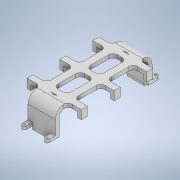
# Autodesk Inventor part: Battery_holder
Saved by Autodesk Inventor 2022 (Build 260153000, 153)
## iProperties
Created: 2023-01-27
Part Number: Battery_holder
Material: Generic
Document SubType Name: Modeling
Designer: Harmonic Ash
Density: 1 g/cm^3
Appearance: Default
Author: Harmonic Ash
Autodesk Inventor part; units mm, degrees
ref_plane "YZ Plane" through (0, 0, 0) normal (1, 0, 0) x (0, 1, 0)
ref_plane "XZ Plane" through (0, 0, 0) normal (0, 1, 0) x (-1, 0, 0)
ref_plane "XY Plane" through (0, 0, 0) normal (0, 0, 1) x (1, 0, 0)
sketch "Sketch1" plane through (0, 0, 0) normal (0, 1, 0) x (-1, 0, 0)
  line L0 (7.7, 0) -> (7.7, 36.5)
  circle A0 centre (7.7, 36.5) radius 0.75
  line L1 (6.2, 30.5) -> (6.2, 36.5)
  circle A1 centre (5.2, 31.5) radius 1
  line L2 (6.2, 30.5) -> (0, 30.5)
  line L3 (0, 30.5) -> (0, 36.5)
  line L4 (0, 36.5) -> (6.2, 36.5)
  line L5 (6.2, 36.5) -> (6.2, 30.5)
  line L6 (7.7, 36.5) -> (0, 36.5)
  line L7 (0, 36.5) -> (0, 0)
  line L8 (0, 0) -> (7.7, 0)
  line L9 (7.7, 0) -> (7.7, 36.5)
  circle A2 centre (7.7, 36.5) radius 1.5
  line L10 (9.2, 36.5) -> (7.7, 36.5)
  line L11 (7.7, 36.5) -> (7.7, 0)
  line L12 (7.7, 0) -> (9.2, 0)
  line L13 (9.2, 0) -> (9.2, 36.5)
  line L14 (6.2, 30.5) -> (0, 30.5)
  line L15 (0, 30.5) -> (0, 33)
  line L16 (0, 33) -> (6.2, 33)
  line L17 (6.2, 33) -> (6.2, 30.5)
  line L18 (9.5, 16) -> (6.5, 16)
  line L19 (6.5, 16) -> (6.5, 0)
  line L20 (6.5, 0) -> (9.5, 0)
  line L21 (9.5, 0) -> (9.5, 16)
  circle A3 centre (8, 16) radius 1.5
  line L22 (0, 0) -> (12.5, 0)
  line L23 (12.5, 0) -> (12.5, 20.5)
  line L24 (12.5, 20.5) -> (0, 20.5)
  line L25 (0, 20.5) -> (0, 0)
  line L26 (0, 20.5) -> (10.2, 20.5)
  line L27 (10.2, 20.5) -> (10.2, 39)
  line L28 (10.2, 39) -> (0, 39)
  line L29 (0, 39) -> (0, 20.5)
  circle A4 centre (7.7, 36.5) radius 2.5
  circle A5 centre (8, 16) radius 4.5
  line L30 (10.2, 20.5) -> (8, 20.5)
  line L31 (8, 20.5) -> (8, 16)
  line L32 (8, 16) -> (10.2, 16)
  line L33 (10.2, 16) -> (10.2, 20.5)
  point P0 (6.2, 31.5)
  point P1 (5.2, 30.5)
  point P2 (12.5, 16)
  point P3 (9.2, 20.337)
  point P4 (7.7, 20.5)
  point P5 (8, 20.5)
  point P6 (7.7, 20.49)
  dimension "d0" = 36.5
  dimension "d2" = 7.7
  dimension "d5" = 1.5
  dimension "d9" = 1.5
  dimension "d12" = 2
  dimension "d13" = 6
  dimension "d14" = 1
  dimension "d15" = 1
  dimension "d16" = 2.5
  dimension "d17" = 3
  dimension "d20" = 9.5
  dimension "d21" = 16
  dimension "d22" = 0
  dimension "d23" = 3
  dimension "d24" = 3
  dimension "d25" = 1
  dimension "d26" = 1
  constraints: 68 end point, 16 parallel, 8 horizontal, 8 perpendicular, 6 centre point, 4 coincident, 3 tangent, 2 point on circle, 1 midpoint, 1 point on line
  measures "d0" distance of L0.start L0.end
  measures "d2" distance from line of L7.end L0
  measures "d5" diameter of A0
  measures "d9" distance between parallel lines of L0 L1
  measures "d12" diameter of A1
  measures "d13" distance between parallel lines of L2 L4
  measures "d14" distance from line of L1 A1.centre
  measures "d15" distance from line of L2 A1.centre
  measures "d16" distance of L14.end L15.end
  measures "d17" distance of L19.end L20.end
  measures "d20" distance between parallel lines of L7 L21
  measures "d21" distance of L18.end L19.end
  measures "d22" distance between parallel lines of L8 L20
  measures "d23" distance between parallel lines of L23 L21
  measures "d24" distance edge to line of A3 L24
  measures "d25" distance between parallel lines of L27 L13
  measures "d26" distance edge to line of A2 L28
extrude "Extrusion1" add sketch "Sketch1" along normal blind 2 contours L8 L19 A5 L0 | L0 A5 L13 L12 | A5 L19 A3 L0 | L0 A3 L13 A5 | L8 L7 L24 L0 A5 L19 | L13 A5 L21 L20 | A5 L0 A3 L19 | L13 A3 L21 A5 | L21 A5 L23 L22 | A5 L31 A3 L0 | L0 L24 A5 | L21 L32 L33 A5 | L7 L2 L1 A4 L0 L24 | A3 L13 A5 L33 L32 | L0 A4 L13 L24 | L24 L13 A5 | A5 L13 A3 L31 | A4 L1 A2 L0 | L0 A2 L13 A4 | A1 L1 L2 | A2 L6 A0 L0 | L0 A0 L10 A2 | A2 L10 A0 L6
sketch "Sketch2" plane through (0, 2, 0) normal (0, 1, 0) x (1, 0, 0)
  line L0 (-5.2, -30.5) -> (0, -30.5) projected
  line L1 (-6.2, -36.5) -> (-6.2, -31.5) projected
  line L2 (0, -30.5) -> (-6.2, -30.5)
  line L3 (-6.2, -30.5) -> (-6.2, -32.5)
  line L4 (-6.2, -32.5) -> (0, -32.5)
  line L5 (0, -32.5) -> (0, -30.5)
  arc A0 (-5.2, -30.5) -> (-6.2, -31.5) centre (-5.2, -31.5) ccw projected
  circle A1 centre (-5.2, -31.5) radius 1
  circle A2 centre (-8, -16) radius 1.5 projected
  circle A3 centre (-8, -16) radius 1.5
  line L6 (-9.5, -16) -> (-6.5, -16)
  line L7 (-6.5, -16) -> (-6.5, 0)
  line L8 (-6.5, 0) -> (-9.5, 0)
  line L9 (-9.5, 0) -> (-9.5, -16)
  point P0 (0, 0)
  dimension "d29" = 2
  constraints: 16 end point, 4 parallel, 2 coincident, 2 horizontal, 2 perpendicular, 1 centre point, 1 horizontal alignment, 1 point on line, 2 other
  measures "d29" distance of L3.end L2.end
extrude "Extrusion2" add sketch "Sketch2" against normal blind 4 contours A1 A0 | L0 L5 L4 A1 | A1 L4 L1 | L6 A2 | A2 L6 | A2 L9 L8 L7
sketch "Sketch4" plane through (0, 2, 0) normal (0, 1, 0) x (1, 0, 0)
  line L0 (0, -30.5) -> (0, 0) projected
  line L1 (-6.5, -29.5) -> (0, -29.5)
  line L2 (0, -29.5) -> (0, 0)
  line L3 (0, 0) -> (-6.5, 0)
  line L4 (-6.5, 0) -> (-6.5, -29.5)
  line L5 (-6.2, -32.5) -> (0, -32.5) projected
  circle A0 centre (-4.5, -27.5) radius 2
  point P0 (-6.5, -27.5)
  point P1 (-4.5, -29.5)
  point P2 (0, -29.5)
  dimension "d32" = 6.5
  dimension "d33" = 3
  dimension "d34" = 2
  dimension "d35" = 2
  constraints: 8 end point, 2 parallel, 1 centre point, 1 horizontal, 1 perpendicular, 1 tangent
  measures "d32" distance between parallel lines of L0 L4
  measures "d33" distance between parallel lines of L1 L5
  measures "d34" distance from line of L4 A0.centre
  measures "d35" distance from line of L1 A0.centre
extrude "Extrusion3" cut sketch "Sketch4" against normal blind 2 contours L1 A0 L4 L3 L0 | A0
mirror "Mirror1" about plane through (0, 0, 0) normal (0, 0, -1) of "Extrusion1", "Extrusion2", "Extrusion3"
mirror "Mirror2" about plane through (0, 0, -30.5) normal (1, 0, 0) of "Extrusion1", "Extrusion2", "Extrusion3", "Mirror1"
sketch "Sketch5" plane through (0, 2, 0) normal (0, 1, 0) x (1, 0, 0)
  line L0 (6.5, 16) -> (6.5, -16) projected
  line L1 (-6.5, -16) -> (-6.5, 16) projected
  line L2 (6.5, 0) -> (-6.5, 0)
  line L3 (-6.5, 0) -> (-6.5, 6)
  line L4 (-6.5, 6) -> (6.5, 6)
  line L5 (6.5, 6) -> (6.5, 0)
  line L6 (6.5, 0) -> (-6.5, 0)
  line L7 (-6.5, 0) -> (-6.5, 3)
  line L8 (-6.5, 3) -> (6.5, 3)
  line L9 (6.5, 3) -> (6.5, 0)
  circle A0 centre (3.5, 6) radius 3
  circle A1 centre (-3.5, 6) radius 3
  point P0 (0, 0)
  point P1 (6.5, 6)
  point P2 (3.5, 3)
  point P3 (-3.5, 3)
  dimension "d38" = 6
  dimension "d41" = 3
  dimension "d42" = 3
  dimension "d43" = 3
  constraints: 16 end point, 4 parallel, 3 point on line, 2 centre point, 2 horizontal, 2 midpoint, 2 perpendicular, 2 tangent
  measures "d38" distance of L2.end L3.end
  measures "d41" distance of L6.end L7.end
  measures "d42" distance of L4.end A0.centre
  measures "d43" distance of L3.end A1.centre
extrude "Extrusion4" add sketch "Sketch5" against normal blind 2 contours L0 L8 A0 | L0 L2 L1 L8 | L8 L1 A1
sketch "Sketch6" plane through (0, 2, 0) normal (0, 1, 0) x (1, 0, 0)
  line L0 (15.25, 30) -> (-15.25, 30)
  line L1 (-15.25, 30) -> (-15.25, -30)
  line L2 (-15.25, -30) -> (15.25, -30)
  line L3 (15.25, -30) -> (15.25, 30)
  point P0 (0, 0)
  dimension "d46" = 60
  dimension "d47" = 30.5
  dimension "d48" = 15.25
  dimension "d49" = 30
  constraints: 8 end point, 2 parallel, 1 horizontal, 1 perpendicular
  measures "d46" distance of L0.end L1.end
  measures "d47" distance of L1.end L2.end
  measures "d48" distance from line of point (0, 0) L3
  measures "d49" distance from line of point (0, 0) L0
extrude "Extrusion5" cut sketch "Sketch6" against normal through all
sketch "Sketch7" plane through (0, 2, 0) normal (0, 1, 0) x (1, 0, 0)
  line L0 (9.2, 30) -> (9.2, 36.5) projected
  line L1 (-9.2, 30) -> (-9.2, 36.5) projected
  line L2 (9.2, 30) -> (-9.2, 30)
  line L3 (-9.2, 30) -> (-9.2, 32.5)
  line L4 (-9.2, 32.5) -> (9.2, 32.5)
  line L5 (9.2, 32.5) -> (9.2, 30)
  point P0 (0, 0)
  dimension "d52" = 2.5
  constraints: 8 end point, 2 parallel, 1 horizontal, 1 perpendicular, 1 point on line
  measures "d52" distance of L2.end L3.end
extrude "Extrusion6" add sketch "Sketch7" along normal blind 12.5
sketch "Sketch8" plane through (-9.2, 0, -36.5) normal (-1, 0, 0) x (0, 0, 1)
  line L0 (6.5, 0) -> (0, 0) projected
  line L1 (6.5, 0) -> (36.5, 0)
  line L2 (36.5, 0) -> (36.5, 15)
  line L3 (36.5, 15) -> (6.5, 15)
  line L4 (6.5, 15) -> (6.5, 0)
  circle A0 centre (10.25, 11.25) radius 3.75
  circle A1 centre (10.25, 11.25) radius 6.25
  line L5 (4, 2) -> (4, 14.5) projected
  line L6 (10.25, 17.5) -> (36.5, 17.5)
  line L7 (36.5, 17.5) -> (36.5, 15)
  line L8 (36.5, 15) -> (10.25, 15)
  line L9 (10.25, 15) -> (10.25, 17.5)
  point P0 (6.5, 6.25)
  point P1 (6.5, 11.25)
  point P2 (10.25, 15)
  dimension "d55" = 15
  dimension "d56" = 7.5
  dimension "d57" = 3.75
  constraints: 16 end point, 4 parallel, 2 horizontal, 2 perpendicular, 1 centre point, 1 coincident, 1 tangent, 1 vertical, 3 other
  measures "d55" distance between parallel lines of L1 L3
  measures "d56" diameter of A0
  measures "d57" distance from line of L3 A0.centre
extrude "Extrusion7" add sketch "Sketch8" against normal up to surface (18.4 mm away) contours A1 L9 L3 L4 | L3 A1 L6 L7 | L4 L3 A0 | L3 L9 A1
sketch "Sketch9" plane through (-9.2, 0, -36.5) normal (-1, 0, 0) x (0, 0, 1)
  arc A0 (10.25, 15) -> (6.5, 11.25) centre (10.25, 11.25) ccw projected
  circle A1 centre (10.25, 11.25) radius 6.25
  line L0 (10.25, 11.25) -> (2.3683, 11.25)
  line L1 (2.3683, 11.25) -> (2.3683, 17.5)
  line L2 (2.3683, 17.5) -> (10.25, 17.5)
  line L3 (10.25, 17.5) -> (10.25, 11.25)
  point P0 (36.5, 0)
  point P1 (4, 11.25)
  constraints: 8 end point, 2 parallel, 1 centre point, 1 coincident, 1 horizontal, 1 perpendicular
extrude "Extrusion8" cut sketch "Sketch9" against normal through all contours A1 L0 L1 L2
sketch "Sketch10" plane through (-9.2, 17.5, 0) normal (0, 1, 0) x (1, 0, 0)
  line L0 (0, 0) -> (18.4, 0) projected
  line L1 (13.7, 0) -> (4.7, 0)
  line L2 (4.7, 0) -> (4.7, 20)
  line L3 (4.7, 20) -> (13.7, 20)
  line L4 (13.7, 20) -> (13.7, 0)
  circle A0 centre (9.2, 20) radius 4.5
  line L5 (0, 0) -> (0, 26.25) projected
  point P0 (9.2, 0)
  dimension "d62" = 9
  dimension "d63" = 20
  dimension "d64" = 4.7
  constraints: 8 end point, 2 parallel, 1 horizontal, 1 midpoint, 1 perpendicular, 1 point on line, 3 other
  measures "d62" distance of L2.end L3.end
  measures "d63" distance of L1.end L2.end
  measures "d64" distance between parallel lines of L5 L2
extrude "Extrusion9" cut sketch "Sketch10" against normal blind 10
mirror "Mirror4" about plane through (-9.2, 17.5, 0) normal (0, 0, 1) of "Extrusion1", "Extrusion2", "Extrusion3", "Mirror1", "Mirror2", "Extrusion4", "Extrusion5", "Extrusion6", "Extrusion7", "Extrusion8", "Extrusion9"
sketch "Sketch11" plane through (-9.2, 17.5, -26.25) normal (0, 1, 0) x (1, 0, 0)
  line L0 (0, 0) -> (0, -52.5) projected
  line L1 (18.4, 0) -> (18.4, -52.5) projected
  line L2 (0, -26.25) -> (18.4, -26.25)
  line L3 (18.4, -26.25) -> (18.4, -24.25)
  line L4 (18.4, -24.25) -> (0, -24.25)
  line L5 (0, -24.25) -> (0, -26.25)
  line L6 (18.4, -24.25) -> (0, -24.25)
  line L7 (0, -24.25) -> (0, -21.25)
  line L8 (0, -21.25) -> (18.4, -21.25)
  line L9 (18.4, -21.25) -> (18.4, -24.25)
  circle A0 centre (10.7, -21.25) radius 3
  circle A1 centre (7.7, -21.25) radius 3
  line L10 (13.7, -6.25) -> (13.7, -46.25) projected
  line L11 (4.7, -46.25) -> (4.7, -6.25) projected
  line L12 (18.4, -24.25) -> (18.4, -21.25)
  line L13 (18.4, -26.25) -> (24.9, -26.25)
  line L14 (24.9, -26.25) -> (24.9, -24.25)
  line L15 (24.9, -24.25) -> (18.4, -24.25)
  line L16 (18.4, -24.25) -> (18.4, -26.25)
  circle A2 centre (21.4, -21.25) radius 3
  point P0 (9.2, -26.25)
  point P1 (13.7, -21.25)
  point P2 (10.7, -24.25)
  point P3 (7.7, -24.25)
  point P4 (4.7, -21.25)
  point P5 (4.7, -26.25)
  point P6 (13.7, -26.25)
  point P7 (21.4, -24.25)
  point P8 (18.4, -21.25)
  dimension "d67" = 2
  dimension "d68" = 3
  dimension "d69" = 3
  dimension "d70" = 3
  dimension "d75" = 6.5
  dimension "d76" = 2
  dimension "d79" = 6
  dimension "d80" = 3
  constraints: 26 end point, 6 parallel, 5 point on line, 3 centre point, 3 horizontal, 3 perpendicular, 2 tangent, 1 midpoint
  measures "d67" distance of L3.end L2.end
  measures "d68" distance of L6.end L7.end
  measures "d69" distance from line of L10 A0.centre
  measures "d70" distance from line of L11 A1.centre
  measures "d75" distance of L15.end L14.end
  measures "d76" distance of L14.end L13.end
  measures "d79" diameter of A2
  measures "d80" distance from line of L1 A2.centre
extrude "Extrusion11" add sketch "Sketch11" against normal blind 2.5 contours A1 L4 L11 | L4 L10 L2 L11 | L10 L4 A0 | A2 L15 L1 | L1 L15 L14 L13
sketch "Sketch12" plane through (15.7, 17.5, 0) normal (1, 0, 0) x (0, 0, -1)
  line L0 (2, 0) -> (5, 0) projected
  line L1 (2, 0) -> (-1, 0)
  line L2 (-1, 0) -> (-1, -6)
  line L3 (-1, -6) -> (2, -6)
  line L4 (2, -6) -> (2, 0)
  point P0 (0, -17.5)
  dimension "d83" = 6
  constraints: 8 end point, 2 parallel, 1 horizontal, 1 perpendicular
  measures "d83" distance of L2.end L1.end
extrude "Extrusion12" add sketch "Sketch12" along normal blind 2.5
mirror "Mirror5" about plane through (15.7, 17.5, 0) normal (0, 0, 1) of "Extrusion11", "Extrusion12"
mirror "Mirror6" about plane through (0, 0, 0) normal (1, 0, 0) of "Extrusion11", "Extrusion12", "Mirror5"
pattern_linear "Rectangular Pattern1" count 3 spacing 22 along (0, 0, -1) of "Extrusion11", "Extrusion12", "Mirror5", "Mirror6" first direction both ways yes
sketch "Sketch13" plane through (-9.2, 0, -36.5) normal (-1, 0, 0) x (0, 0, 1)
  arc A0 (9.5, 17.4548) -> (4, 11.25) centre (10.25, 11.25) ccw projected
  circle A1 centre (10.25, 11.25) radius 6.25
  circle A2 centre (10.25, 11.25) radius 3.75
  line L0 (10.25, 11.25) -> (4, 11.25)
  line L1 (4, 11.25) -> (4, 17.5)
  line L2 (4, 17.5) -> (10.25, 17.5)
  line L3 (10.25, 17.5) -> (10.25, 11.25)
  point P0 (36.5, 0)
  point P1 (4, 11.25)
  point P2 (9.5, 17.4548)
  constraints: 8 end point, 2 centre point, 2 coincident, 2 parallel, 1 horizontal, 1 perpendicular
extrude "Extrusion13" cut sketch "Sketch13" along normal through all both and the other way through all contours A0 L1 L2 A1
equation "\"d2\" = 0.5 * d1"
equation "\"d48\" = 0.5 * d47"
equation "\"d49\" = 0.5 * d46"
equation "\"d57\" = 0.5 * d56"
equation "\"d1\" = 15.4"
body "Solid1"
